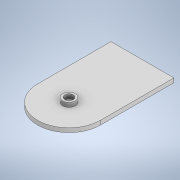
# Autodesk Inventor part: daodwaw
Saved by Autodesk Inventor 2020 (Build 240168000, 168)
## iProperties
Created: 2020-01-27
Part Number: daodwaw
Material: Generic
Document SubType Name: Modeling
Designer: maple
Density: 1 g/cm^3
Appearance: Default
Author: maple
Autodesk Inventor part; units mm, degrees
ref_plane "YZ Plane" through (0, 0, 0) normal (1, 0, 0) x (0, 1, 0)
ref_plane "XZ Plane" through (0, 0, 0) normal (0, 1, 0) x (-1, 0, 0)
ref_plane "XY Plane" through (0, 0, 0) normal (0, 0, 1) x (1, 0, 0)
sketch "Sketch1" plane through (0, 0, 0) normal (0, 1, 0) x (-1, 0, 0)
  line L0 (0, 0) -> (-76.2, 0)
  line L1 (-76.2, 0) -> (-76.2, -127)
  line L2 (-76.2, -127) -> (0, -127)
  line L3 (0, -127) -> (0, 0)
  dimension "d0" = 76.2
  dimension "d1" = 127
  constraints: 8 end point, 2 parallel, 1 horizontal, 1 perpendicular
  measures "d0" distance of L2.end L1.end
  measures "d1" distance of L1.end L0.end
extrude "Extrusion1" add sketch "Sketch1" along normal blind 5.08
fillet "Fillet1" radius 38.1 2 edges at (76.2, 2.54, 0) (0, 2.54, 0)
sketch "Sketch2" plane through (0, 5.08, 0) normal (0, 1, 0) x (1, 0, 0)
  arc A0 (0, 38.1) -> (76.2, 38.1) centre (38.1, 38.1) ccw projected
  line L0 (38.1, 0) -> (38.1, 38.1)
  circle A1 centre (38.1, 38.1) radius 7.62
  circle A2 centre (38.1, 38.1) radius 5.08
  point P0 (0, 0)
  dimension "d5" = 15.24
  dimension "d6" = 10.16
  constraints: 2 centre point, 2 coincident, 2 end point, 1 point on circle, 1 vertical
  measures "d5" diameter of A1
  measures "d6" diameter of A2
extrude "Extrusion2" add sketch "Sketch2" along normal blind 5.08
body "Solid1"
